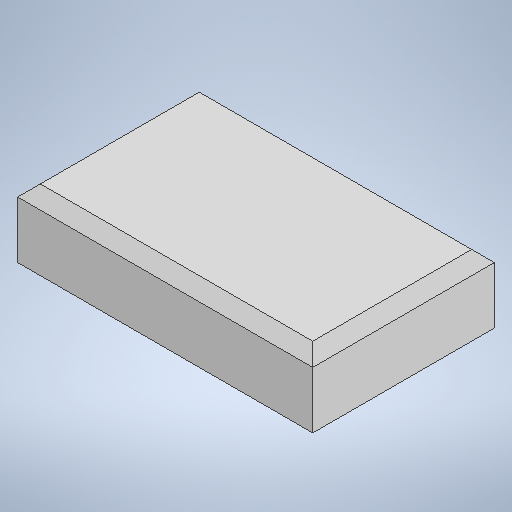
# Autodesk Inventor part: block
Saved by Autodesk Inventor 2025.1 (Build 291241000, 241)
## iProperties
Created: 2024-09-13
Part Number: block
Material: Generisch
Document SubType Name: Modeling
Designer: ffogue
Density: 1 g/cm^3
Appearance: Vorgabe
Author: ffogue
Autodesk Inventor part; units mm, degrees
ref_plane "YZ Plane" through (0, 0, 0) normal (1, 0, 0) x (0, 1, 0)
ref_plane "XZ Plane" through (0, 0, 0) normal (0, 1, 0) x (-1, 0, 0)
ref_plane "XY Plane" through (0, 0, 0) normal (0, 0, 1) x (1, 0, 0)
sketch "Sketch1" plane through (0, 0, 0) normal (0, 0, 1) x (1, 0, 0)
  line L0 (-65, -40) -> (65, -40)
  line L1 (65, -40) -> (65, 40)
  line L2 (65, 40) -> (-65, 40)
  line L3 (-65, 40) -> (-65, -40)
  line L4 (-65, -40) -> (65, 40) construction
  line L5 (65, -40) -> (-65, 40) construction
  point P0 (0, 0)
  dimension "d0" = 80
  dimension "d1" = 130
  constraints: 12 end point, 2 midpoint, 2 parallel, 1 horizontal, 1 perpendicular
  measures "d0" distance of L2.end L0.start
  measures "d1" distance of L1.end L2.end
extrude "Extrusion1" add sketch "Sketch1" along normal blind 30
sketch "Sketch2" plane through (0, 0, 30) normal (0, 0, 1) x (1, 0, 0)
  line L0 (-65, -40) -> (65, -40) projected
  line L1 (65, -40) -> (65, 40) projected
  line L2 (65, 40) -> (-65, 40) projected
  point P0 (0, 0)
  point P1 (0, 40)
  constraints: 1 midpoint
hole "Hole1" at (0, 40, 30) direction (0, 0, -1) diameter 9 depth 30
chamfer "Chamfer1" distance 5 angle 45 5 edges at (34.75, 40, 30) (-34.75, 40, 30) (65, 0, 30) (0, -40, 30) (-65, 0, 30)
body "Solid1"
